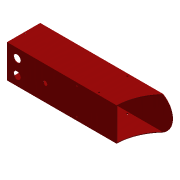
# Autodesk Inventor part: Case
Saved by Autodesk Inventor 2015 (Build 190159000, 159)
## iProperties
Created: 2015-01-07
Part Number: Case
Material: Všeobecné
Document SubType Name: Modeling
Designer: Michal
Density: 1 g/cm^3
Appearance: Červená
Author: Michal
Autodesk Inventor part; units mm, degrees
ref_plane "YZ Plane" through (0, 0, 0) normal (1, 0, 0) x (0, 1, 0)
ref_plane "XZ Plane" through (0, 0, 0) normal (0, 1, 0) x (-1, 0, 0)
ref_plane "XY Plane" through (0, 0, 0) normal (0, 0, 1) x (1, 0, 0)
sketch "Náčrt1" plane through (0, 0, 0) normal (1, 0, 0) x (0, 1, 0)
  line L0 (0, 0) -> (100, 0)
  line L1 (100, 0) -> (100, -100)
  line L2 (100, -100) -> (0, -100)
  line L3 (0, -100) -> (0, 0)
  line L4 (98, -2) -> (2, -2)
  line L5 (2, -2) -> (2, -98)
  line L6 (2, -98) -> (98, -98)
  line L7 (98, -98) -> (98, -2)
  dimension "d0" = 100
  dimension "d1" = 100
  dimension "d2" = 2
  constraints: 16 end point, 4 parallel, 2 perpendicular, 1 horizontal, 3 other
  measures "d0" distance of L1.end L2.end
  measures "d1" distance of L0.end L1.end
  measures "d2" distance between parallel lines of L0 L4
extrude "Vysunutí1" add sketch "Náčrt1" along normal blind 370
sketch "Náčrt4" plane through (0, 0, 0) normal (0, 0, 1) x (1, 0, 0)
  circle A0 centre (479.9456, -4.039) radius 150
  line L0 (0, 0) -> (0, 100) projected
  line L1 (0, 0) -> (370, 0) projected
  line L2 (370, 100) -> (370, 0) projected
  line L3 (0, 100) -> (370, 100) projected
  line L4 (330, 0) -> (370, 0)
  line L5 (370, 0) -> (370, 98)
  dimension "d16" = 300
  dimension "d17" = 2
  dimension "d18" = 330
  constraints: 4 end point, 2 point on circle, 2 point on line, 1 centre point, 1 collinear, 1 horizontal
  measures "d16" diameter of A0
  measures "d17" distance from line of L3 L5.end
  measures "d18" distance of point (0, 0) L4.start
extrude "Vysunutí4" cut sketch "Náčrt4" against normal through all contours L2 L1 A0 picked at (366.6963, 61.3839)
sketch "Náčrt5" plane through (0, 100, 0) normal (0, 1, 0) x (1, 0, 0)
  line L0 (0, 0) -> (0, 100) projected
  line L1 (0, 0) -> (370, 0) projected
  line L2 (370, 100) -> (370, 0) projected
  line L3 (0, 100) -> (370, 100) projected
  arc A0 (370, 0) -> (370, 100) centre (343.3333, 50) ccw
  point P0 (400, 50)
  dimension "d21" = 30
  constraints: 3 point on circle, 1 centre point
  measures "d21" distance from line of point (400, 50) L2
extrude "Vysunutí5" add sketch "Náčrt5" against normal blind 2 contours L2 A0
sketch "Náčrt11" plane through (0, 0, -100) normal (0, -1, 0) x (1, 0, 0)
  line L0 (330, 0) -> (330, 100) projected
  line L1 (0, 100) -> (330, 100) projected
  line L2 (0, 0) -> (0, 100) projected
  line L3 (0, 0) -> (330, 0) projected
  circle A0 centre (115, 50) radius 6.25
  dimension "d57" = 12.5
  dimension "d58" = 115
  constraints: 1 centre point
  measures "d57" diameter of A0
  measures "d58" distance from line of L2 A0.centre
extrude "Vysunutí11" cut sketch "Náčrt11" against normal blind 5 contours A0
sketch "Náčrt12" plane through (0, 0, -100) normal (0, -1, 0) x (1, 0, 0)
  circle A0 centre (115, 50) radius 6.25 projected
  line L0 (330, 0) -> (330, 100) projected
  line L1 (0, 100) -> (330, 100) projected
  line L2 (0, 0) -> (0, 100) projected
  line L3 (0, 0) -> (330, 0) projected
  circle A1 centre (210, 90) radius 2.25
  circle A2 centre (210, 10) radius 2.25
  dimension "d61" = 4.5
  dimension "d62" = 4.5
  dimension "d63" = 10
  dimension "d64" = 10
  dimension "d65" = 210
  dimension "d66" = 210
  constraints: 2 centre point
  measures "d61" diameter of A1
  measures "d62" diameter of A2
  measures "d63" distance from line of L1 A1.centre
  measures "d64" distance from line of L3 A2.centre
  measures "d65" distance from line of L2 A2.centre
  measures "d66" distance from line of L2 A1.centre
extrude "Vysunutí12" cut sketch "Náčrt12" against normal blind 10 contours A1 | A2
sketch "Náčrt13" plane through (0, 0, -100) normal (0, -1, 0) x (1, 0, 0)
  circle A0 centre (210, 90) radius 2.25 projected
  circle A1 centre (210, 10) radius 2.25 projected
  circle A2 centre (115, 50) radius 6.25 projected
  line L0 (330, 0) -> (330, 100) projected
  line L1 (0, 100) -> (330, 100) projected
  line L2 (0, 0) -> (0, 100) projected
  line L3 (0, 0) -> (330, 0) projected
  circle A3 centre (30, 72) radius 11
  circle A4 centre (30, 28) radius 11
  dimension "d69" = 22
  dimension "d70" = 22
  dimension "d71" = 28
  dimension "d72" = 30
  dimension "d73" = 30
  dimension "d74" = 28
  constraints: 2 centre point
  measures "d69" diameter of A3
  measures "d70" diameter of A4
  measures "d71" distance from line of L1 A3.centre
  measures "d72" distance from line of A3.centre L2
  measures "d73" distance from line of L2 A4.centre
  measures "d74" distance from line of L3 A4.centre
extrude "Vysunutí13" cut sketch "Náčrt13" against normal up to surface (2 mm away) contours A3 | A4
sketch "Náčrt14" plane through (0, 0, -100) normal (0, 0, -1) x (-1, 0, 0)
  arc A0 (-330, 0) -> (-370, 98) centre (-479.9456, -4.039) ccw projected
  line L0 (0, 0) -> (-330, 0) projected
  line L1 (0, 100) -> (0, 0) projected
  line L2 (0, 100) -> (-370, 100) projected
  line L3 (-370, 98) -> (-370, 100) projected
  circle A1 centre (-270, 7.5) radius 2.25
  circle A2 centre (-270, 92.5) radius 2.25
  circle A3 centre (-5, 50) radius 1.75
  dimension "d77" = 270
  dimension "d78" = 4.5
  dimension "d79" = 4.5
  dimension "d80" = 270
  dimension "d81" = 3.5
  dimension "d82" = 5
  dimension "d83" = 50
  dimension "d86" = 85
  dimension "d87" = 7.5
  constraints: 3 centre point
  measures "d77" distance from line of L1 A1.centre
  measures "d78" diameter of A1
  measures "d79" diameter of A2
  measures "d80" distance from line of L1 A2.centre
  measures "d81" diameter of A3
  measures "d82" distance from line of L1 A3.centre
  measures "d83" distance from line of L0 A3.centre
  measures "d86" distance of A1.centre A2.centre
  measures "d87" distance from line of L2 A2.centre
extrude "Vysunutí14" cut sketch "Náčrt14" against normal through all contours A1 | A2 | A3
